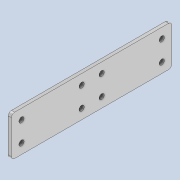
# Autodesk Inventor part: 2x4 2020 Extrusion Gusset Connector
Saved by Autodesk Inventor 2022 (Build 260153000, 153)
## iProperties
Created: 2021-10-23
Part Number: 2x4 2020 Extrusion Gusset Connector
Material: Generic
Document SubType Name: Modeling
Designer: Coy
Density: 1 g/cm^3
Appearance: Machined - Aluminum
Author: Coy
Autodesk Inventor part; units mm, degrees
ref_plane "YZ Plane" through (0, 0, 0) normal (1, 0, 0) x (0, 1, 0)
ref_plane "XZ Plane" through (0, 0, 0) normal (0, 1, 0) x (-1, 0, 0)
ref_plane "XY Plane" through (0, 0, 0) normal (0, 0, 1) x (1, 0, 0)
sketch "Sketch1" plane through (0, 0, 0) normal (1, 0, 0) x (0, 1, 0)
  line L0 (0, 0) -> (40, 0)
  line L1 (40, 0) -> (40, 160)
  line L2 (40, 160) -> (0, 160)
  line L3 (0, 160) -> (0, 0)
  line L4 (40, 80) -> (0, 80) construction
  line L5 (30, 70) -> (10, 70) construction
  line L6 (10, 70) -> (10, 10) construction
  line L7 (10, 10) -> (30, 10) construction
  line L8 (30, 10) -> (30, 70) construction
  line L9 (30, 70) -> (40, 70) construction
  line L10 (30, 70) -> (30, 80) construction
  line L11 (10, 10) -> (0, 10) construction
  line L12 (10, 10) -> (10, 0) construction
  circle A0 centre (30, 70) radius 2.6
  circle A1 centre (30, 10) radius 2.6
  circle A2 centre (10, 10) radius 2.6
  circle A3 centre (10, 70) radius 2.6
  circle A4 centre (30, 90) radius 2.6
  circle A5 centre (30, 150) radius 2.6
  circle A6 centre (10, 150) radius 2.6
  circle A7 centre (10, 90) radius 2.6
  dimension "d0" = 40
  dimension "d1" = 160
  dimension "d2" = 20
  dimension "d3" = 60
  dimension "d4" = 5.2
  dimension "d5" = 5.2
  dimension "d6" = 5.2
  dimension "d7" = 5.2
  constraints: 26 end point, 8 centre point, 6 parallel, 6 perpendicular, 4 coincident, 4 point on line, 4 symmetric about line, 2 horizontal, 2 midpoint, 4 other
  measures "d0" distance of L2.end L1.end
  measures "d1" distance of L1.end L0.end
  measures "d2" distance of L5.start L5.end
  measures "d3" distance of L7.end L5.start
  measures "d4" diameter of A0
  measures "d5" diameter of A1
  measures "d6" diameter of A2
  measures "d7" diameter of A3
extrude "Extrusion1" add sketch "Sketch1" against normal blind 3.175
fillet "Fillet1" radius 3.175 4 edges at (-1.5875, 40, 160) (-1.5875, 0, 160) (-1.5875, 40, 0) (-1.5875, 0, 0)
equation "\"d5\" = d4"
equation "\"d6\" = d4"
equation "\"d7\" = d4"
body "Solid1"
